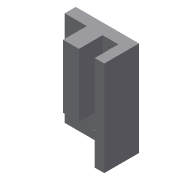
# Autodesk Inventor part: base
Saved by Autodesk Inventor 2022 (Build 260148000, 148)
## iProperties
Shininess: 64.0
Length Units: 11269
Angle Units: 11279
Time Units: 11290
Mass Units: 11283
Length Display Precision: 3
Angle Display Precision: 2
Created: 2001-12-31
Part Number: base
Document SubType Name: Modeling
Designer: Administrator
Density: 1 g/cm^3
Material: Generic
Appearance: Default
Density: 0.0
Volumn: 0.0
Area: 0.0
PropertySet Name: Model Information
Control State: 0
Master: False
Checked Out: False
Author: Administrator
Autodesk Inventor part; units mm, degrees
ref_plane "YZ Plane" through (0, 0, 0) normal (1, 0, 0) x (0, 1, 0)
ref_plane "XZ Plane" through (0, 0, 0) normal (0, 1, 0) x (-1, 0, 0)
ref_plane "XY Plane" through (0, 0, 0) normal (0, 0, 1) x (1, 0, 0)
sketch "Sketch1" plane through (0, 0, 0) normal (0, 0, 1) x (1, 0, 0)
  line L0 (-33.7638, 59.8408) -> (17.0362, 59.8408)
  line L1 (17.0362, 59.8408) -> (17.0362, -16.3592)
  line L2 (17.0362, -16.3592) -> (-33.7638, -16.3592)
  line L3 (-33.7638, -16.3592) -> (-33.7638, 59.8408)
  dimension "d0" = 50.8
  dimension "d1" = 76.2
  constraints: 8 end point, 2 parallel, 1 horizontal, 1 perpendicular
  measures "d0" distance of L1.end L2.end
  measures "d1" distance of L2.end L0.start
extrude "Extrusion1" add sketch "Sketch1" along normal blind 8.89
sketch "Sketch2" plane through (0, 0, 8.89) normal (0, 0, 1) x (1, 0, 0)
  line L0 (17.0362, 59.8408) -> (17.0362, -16.3592) projected
  line L1 (-33.7638, 59.8408) -> (17.0362, 59.8408) projected
  line L2 (17.0362, -16.3592) -> (-33.7638, -16.3592) projected
  line L3 (9.4162, 59.8408) -> (9.4162, -16.3592)
  dimension "d4" = 7.62
  constraints: 2 end point, 2 perpendicular, 2 point on line
  measures "d4" distance of L3.start L0.start
extrude "Extrusion2" add sketch "Sketch2" along normal blind 19.05
sketch "Sketch3" plane through (0, 0, 8.89) normal (0, 0, 1) x (1, 0, 0)
  point P0 (9.4162, -16.3592)
  point P1 (-33.7638, -16.3592)
  point P2 (-9.6338, -8.7392)
  point P3 (-25.6982, -1.1192)
  dimension "d7" = 19.05
  dimension "d8" = 7.62
  dimension "d9" = 17.78
  dimension "d10" = 15.24
  measures "d7" horizontal distance of point (9.416, -16.359) point (-9.634, -8.739)
  measures "d8" vertical distance of point (-33.764, -16.359) point (-9.634, -8.739)
  measures "d9" distance of point (-9.634, -8.739) point (-25.698, -1.119)
  measures "d10" vertical distance of point (-33.764, -16.359) point (-25.698, -1.119)
hole "Hole1" at (-9.6338, -8.7392, 8.89) at (-25.6982, -1.1192, 8.89) direction (0, 0, -1) diameter 2.54 depth 12.7 tip angle 118
sketch "Sketch4" plane through (0, 0, 8.89) normal (0, 0, 1) x (1, 0, 0)
  line L0 (9.4162, -16.3592) -> (9.4162, 59.8408) projected
  line L1 (-33.7638, 59.8408) -> (9.4162, 59.8408) projected
  line L2 (-15.9838, 59.8408) -> (-15.9838, 9.0408)
  line L3 (-15.9838, 9.0408) -> (-3.2838, 9.0408)
  line L4 (-3.2838, 9.0408) -> (-3.2838, 59.8408)
  dimension "d18" = 12.7
  dimension "d19" = 12.7
  dimension "d22" = 50.8
  constraints: 6 end point, 2 point on line, 1 horizontal, 1 parallel, 1 perpendicular
  measures "d18" distance of L0.end L4.end
  measures "d19" distance of L4.end L2.start
  measures "d22" distance of L2.start L2.end
extrude "Extrusion3" add sketch "Sketch4" along normal up to surface (19.05 mm away)
sketch "Sketch5" plane through (0, 0, 8.89) normal (0, 0, 1) x (1, 0, 0)
  line L0 (-3.2838, 59.8408) -> (9.4162, 59.8408) projected
  line L1 (-3.2838, 59.8408) -> (-3.2838, 9.0408) projected
  circle A0 centre (3.0662, 53.4908) radius 2.074
  dimension "d24" = 6.35
  dimension "d25" = 6.35
  constraints: 1 centre point
  measures "d24" distance from line of L1 A0.centre
  measures "d25" distance from line of L0 A0.centre
extrude "Extrusion4" cut sketch "Sketch5" against normal up to next
body "Solid1"
